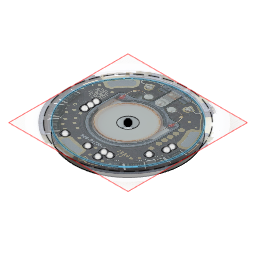
airtag-beta-base (Autodesk Fusion 360 design; units mm, degrees)
Autodesk Fusion 360 part; units mm, degrees
sketch "Sketch1" plane through (0, 0, 0) normal (0, 1, 0) x (1, 0, 0)
  circle A0 centre (0, 0) radius 13 construction
  circle A1 centre (0, 0) radius 11.8004
  point P0 (-7.45, 0.5)
  point P1 (-7.45, -0.75)
  point P2 (-7.4065, -2.039)
  point P3 (9.3586, 0.2369)
  point P4 (9.3586, -0.9412)
  point P5 (8.3, -3.7)
  point P6 (-4.8, -8.9)
  point P7 (-0.0017, -8.7426)
  point P8 (4.1864, -8.1521)
  point P9 (2.9094, -8.1521)
  point P10 (3.1291, -9.6832)
  dimension "d1" = 26
  constraint coincident A0.centre A1.centre
  measures "d1" diameter of A0
extrude "Extrude1" add sketch "Sketch1" against normal blind 2
hole "Hole1" at (-7.45, 0, -0.5) at (-7.45, 0, 0.75) at (-7.4065, 0, 2.039) at (-4.8, 0, 8.9) at (-0.0017, 0, 8.7426) at (2.9094, 0, 8.1521) at (3.1291, 0, 9.6832) at (4.1864, 0, 8.1521) at (8.3, 0, 3.7) at (9.3586, 0, 0.9412) at (9.3586, 0, -0.2369) direction (0, -1, 0) diameter 1.6 depth 5.5 tip angle 118
hole "Hole2" at (0, 0, 0) direction (0, -1, 0) diameter 3.5 depth 5.5 tip angle 118
